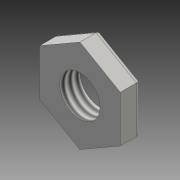
# Autodesk Inventor part: 螺母
Saved by Autodesk Inventor 2016 (Build 200138000, 138)
## iProperties
Created: 2019-05-19
Part Number: 螺母
Material: 常规
Document SubType Name: Modeling
Designer: oldboy
Density: 1 g/cm^3
Appearance: 默认
Author: oldboy
Autodesk Inventor part; units mm, degrees
ref_plane "YZ Plane" through (0, 0, 0) normal (1, 0, 0) x (0, 1, 0)
ref_plane "XZ Plane" through (0, 0, 0) normal (0, 1, 0) x (-1, 0, 0)
ref_plane "XY Plane" through (0, 0, 0) normal (0, 0, 1) x (1, 0, 0)
sketch "草图1" plane through (0, 0, 0) normal (0, 1, 0) x (-1, 0, 0)
  circle A0 centre (0, 0) radius 2
  line L0 (4, -2.3094) -> (0, -4.6188)
  line L1 (0, -4.6188) -> (-4, -2.3094)
  line L2 (-4, -2.3094) -> (-4, 2.3094)
  line L3 (-4, 2.3094) -> (0, 4.6188)
  line L4 (0, 4.6188) -> (4, 2.3094)
  line L5 (4, 2.3094) -> (4, -2.3094)
  point P0 (4, 0)
  dimension "d0" = 4
  constraints: 12 end point, 1 centre point, 1 coincident, 1 midpoint, 13 other
  measures "d0" diameter of A0
extrude "拉伸1" add sketch "草图1" along normal blind 2
fillet "圆角1" radius 0.4 6 edges at (-2, 2, 3.4641) (-4, 2, 0) (-2, 2, -3.4641) (2, 2, -3.4641) (4, 2, 0) (2, 2, 3.4641)
thread "螺纹1" size "M4x0.7" class "6H" standard "ANSI Metric M Profile" full length
